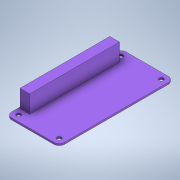
# Autodesk Inventor part: raspberry
Saved by Autodesk Inventor 2021 (Build 250183000, 183)
## iProperties
Created: 2021-02-15
Part Number: raspberry
Material: Generic
Document SubType Name: Modeling
Designer: lobato
Density: 1 g/cm^3
Appearance: Default
Author: lobato
Autodesk Inventor part; units mm, degrees
ref_plane "YZ Plane" through (0, 0, 0) normal (1, 0, 0) x (0, 1, 0)
ref_plane "XZ Plane" through (0, 0, 0) normal (0, 1, 0) x (-1, 0, 0)
ref_plane "XY Plane" through (0, 0, 0) normal (0, 0, 1) x (1, 0, 0)
sketch "Sketch1" plane through (0, 0, 0) normal (0, 1, 0) x (-1, 0, 0)
  line L0 (15, 32.5) -> (-15, 32.5)
  line L1 (-15, 32.5) -> (-15, -32.5)
  line L2 (-15, -32.5) -> (15, -32.5)
  line L3 (15, -32.5) -> (15, 32.5)
  line L4 (15, 32.5) -> (-15, -32.5) construction
  line L5 (-15, 32.5) -> (15, -32.5) construction
  line L6 (11.5, 29) -> (-11.5, 29) construction
  line L7 (-11.5, 29) -> (-11.5, -29) construction
  line L8 (-11.5, -29) -> (11.5, -29) construction
  line L9 (11.5, -29) -> (11.5, 29) construction
  line L10 (11.5, 29) -> (-11.5, -29) construction
  line L11 (-11.5, 29) -> (11.5, -29) construction
  circle A0 centre (11.5, 29) radius 1.25
  circle A1 centre (11.5, -29) radius 1.25
  circle A2 centre (-11.5, -29) radius 1.25
  circle A3 centre (-11.5, 29) radius 1.25
  point P0 (0, 0)
  dimension "d0" = 30
  dimension "d1" = 65
  dimension "d2" = 23
  dimension "d3" = 58
  dimension "d4" = 2.5
  dimension "d5" = 2.5
  dimension "d6" = 2.5
  dimension "d7" = 2.5
  constraints: 24 end point, 4 centre point, 4 coincident, 4 midpoint, 4 parallel, 2 horizontal, 2 perpendicular
  measures "d0" distance of L2.end L1.end
  measures "d1" distance of L1.end L0.end
  measures "d2" distance of L8.end L7.end
  measures "d3" distance of L7.end L6.end
  measures "d4" diameter of A0
  measures "d5" diameter of A1
  measures "d6" diameter of A2
  measures "d7" diameter of A3
extrude "Extrusion1" add sketch "Sketch1" along normal blind 1
fillet "Fillet1" radius 3 4 edges at (-15, 0.5, 32.5) (15, 0.5, 32.5) (15, 0.5, -32.5) (-15, 0.5, -32.5)
sketch "Sketch2" plane through (0, 1, 0) normal (0, 1, 0) x (1, 0, 0)
  line L0 (-14.25, -25.5) -> (-8.75, -25.5)
  line L1 (-8.75, -25.5) -> (-8.75, 25.5)
  line L2 (-8.75, 25.5) -> (-14.25, 25.5)
  line L3 (-14.25, 25.5) -> (-14.25, -25.5)
  line L4 (-14.25, -25.5) -> (-8.75, 25.5) construction
  line L5 (-8.75, -25.5) -> (-14.25, 25.5) construction
  line L6 (-15, 29.5) -> (-15, -29.5) projected
  point P0 (0, 0)
  point P1 (-11.5, 0)
  dimension "d11" = 5.5
  dimension "d12" = 51
  dimension "d13" = 3.5
  constraints: 12 end point, 2 midpoint, 2 parallel, 1 horizontal, 1 perpendicular
  measures "d11" distance of L2.end L1.end
  measures "d12" distance of L1.end L0.end
  measures "d13" distance from line of L6 point (-11.5, 0)
extrude "Extrusion2" add sketch "Sketch2" along normal blind 10 and the other way blind 3
body "Solid1"
